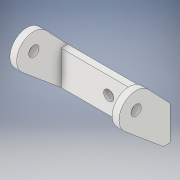
# Autodesk Inventor part: Neck
Saved by Autodesk Inventor 2017 SP1 (Build 210196100, 196)
## iProperties
Created: 2018-02-11
Part Number: Neck
Material: ABS Plastic
Document SubType Name: Modeling
Designer: Zach
Density: 1.06 g/cm^3
Appearance: CR White
Author: Zach
Autodesk Inventor part; units mm, degrees
ref_plane "YZ Plane" through (0, 0, 0) normal (1, 0, 0) x (0, 1, 0)
ref_plane "XZ Plane" through (0, 0, 0) normal (0, 1, 0) x (-1, 0, 0)
ref_plane "XY Plane" through (0, 0, 0) normal (0, 0, 1) x (1, 0, 0)
sketch "Sketch1" plane through (0, 0, 0) normal (0, 0, 1) x (1, 0, 0)
  line L0 (0, 0) -> (32, 0)
  line L1 (32, 0) -> (32, 10)
  line L2 (32, 10) -> (0, 10)
  line L3 (0, 10) -> (0, 0)
  dimension "d0" = 32
  dimension "d1" = 10
  constraints: 8 end point, 2 parallel, 1 horizontal, 1 perpendicular
  measures "d0" distance of L2.end L1.end
  measures "d1" distance of L1.end L0.end
extrude "Extrusion1" add sketch "Sketch1" along normal blind 2
sketch "Sketch2" plane through (0, 0, 2) normal (0, 0, 1) x (1, 0, 0)
  line L0 (32, 10) -> (0, 10) projected
  line L1 (0, 10) -> (0, 0) projected
  circle A0 centre (16, 5) radius 1.5
  point P0 (16, 10)
  point P1 (0, 5)
  dimension "d4" = 3
  constraints: 2 midpoint, 1 centre point, 1 horizontal alignment, 1 vertical alignment
  measures "d4" diameter of A0
extrude "Extrusion2" cut sketch "Sketch2" against normal through all
sketch "Sketch3" plane through (32, 0, 0) normal (1, 0, 0) x (0, 0, -1)
  circle A0 centre (-10, 13.2398) radius 5 construction
  line L0 (0, 0) -> (0, 10) projected
  line L1 (-2, 10) -> (-2, 0) projected
  line L2 (-2, 0) -> (-13.2139, 9.4096)
  line L3 (0, 10) -> (-6.3819, 16.6909)
  arc A1 (-6.3819, 16.6909) -> (-13.2139, 9.4096) centre (-10, 13.2398) ccw
  circle A2 centre (-10, 13.2398) radius 1.5
  line L4 (0, 10) -> (-2, 10) projected
  dimension "d7" = 10
  dimension "d8" = 10
  dimension "d9" = 50
  dimension "d10" = 3
  constraints: 4 end point, 4 point on circle, 4 tangent, 3 centre point, 1 coincident
  measures "d7" diameter of A0
  measures "d8" distance from line of L0 A0.centre
  measures "d9" angle of L2 L1
  measures "d10" diameter of A2
extrude "Extrusion3" add sketch "Sketch3" against normal blind 2
sketch "Sketch4" plane through (0, 0, 0) normal (-1, 0, 0) x (0, 0, 1)
  circle A0 centre (10, 13.2398) radius 1.5 projected
  line L0 (6.3819, 16.6909) -> (0, 10) projected
  line L1 (2, 10) -> (0, 10) projected
  line L2 (2, 0) -> (2, 10) projected
  line L3 (2, 0) -> (13.2139, 9.4096) projected
  arc A1 (13.2139, 9.4096) -> (6.3819, 16.6909) centre (10, 13.2398) ccw projected
  point P0 (0, 0)
extrude "Extrusion4" add sketch "Sketch4" against normal blind 2
body "Solid1"
